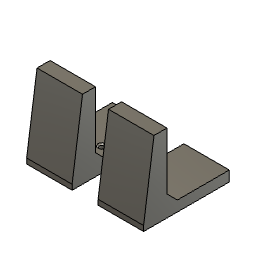
wordclock_standfuss_v2 (Autodesk Fusion 360 design; units mm, degrees)
Autodesk Fusion 360 part; units mm, degrees
other "Grundnetzelement1"
sketch "Skizze1" plane through (20, 30, 0) normal (1, 0, 0) x (0, 1, 0)
other "Netzschnitt1"
sketch "Skizze2" plane through (-10, 30, 0) normal (1, 0, 0) x (0, 1, 0)
  line L0 (-30, 33) -> (-26, 33)
  line L1 (-26, 33) -> (-26, -33)
  line L2 (-26, -33) -> (-30, -33)
  line L3 (-30, -33) -> (-30, 33)
  line L4 (-26, 15) -> (30, 15)
  line L5 (30, 15) -> (30, 25)
  line L6 (30, 25) -> (-26, 25)
  line L7 (-26, 25) -> (-26, 15)
  line L8 (30, 25) -> (-26, 33)
  line L9 (-26, 33) -> (-27.26, 24.18)
  line L10 (-27.26, 24.18) -> (28.74, 16.18)
  line L11 (28.74, 16.18) -> (30, 25)
  constraint horizontal L0
  constraint vertical L1
  constraint horizontal L2
  constraint vertical L3
  constraint horizontal L4
  constraint vertical L5
  constraint horizontal L6
  constraint vertical L7
  constraint coincident L1 L4.start
  constraint perpendicular L8 L9
  constraint parallel L8 L10
  constraint parallel L9 L11
other "Netzschnitt2"
sketch "Skizze3" plane through (-10, 1, 0) normal (0, 1, 0) x (-1, 0, 0)
  circle A0 centre (-10, 0) radius 2
other "Netzschnitt3"
extrude "Extrusion1" add sketch "Skizze2" along normal blind 20 makes body 1
extrude "Extrusion2" add 1 faces at (-10, 22.6667, 24.3333) along direction (-1, 0, 0) blind 20 on bodies 1 bodies 1
extrude "Extrusion3" cut sketch "Skizze3" along normal blind 4 bodies 1
extrude "Extrusion4" cut 1 faces at (-0.6006, 1, 0.0905) along direction (0, -1, 0) blind 9 on bodies 1 bodies 1
extrude "Extrusion5" add 1 faces at (-20.637, 4, -6.1965) along direction (0, 1, 0) blind 4 on bodies 1 bodies 1
chamfer "Fase1" distance 8 angle 45 1 edges at (-10, 8, 15) on bodies 1
chamfer "Fase2" distance 1 angle 45 1 edges at (1.8647, 8, 0.7232) on bodies 1
extrude "Extrusion6" cut 1 faces at (-30, 26.6667, 24.3333) along direction (1, 0, 0) blind 5 on bodies 1 bodies 1
ref_plane "Arbeitsebene1" through (20, 30, 0) normal (1, 0, 0) x (0, 0, -1)
mirror "Spiegeln1" about plane through (20, 30, 0) normal (1, 0, 0) of bodies 1 makes body 2
copy_body "Körper->Berechn1" bodies 2 removing the originals makes body 3 in component "standfuss_v2_mirrored"
copy_body "Körper->Berechn2" bodies 1 removing the originals makes body 4 in component "standfuss_v2_normal"
component "standfuss_v2_mirrored" placed x (1, 0, 0) y (0, 1, 0) z (0, 0, 1) at (0, 0, 0)
component "standfuss_v2_normal" placed x (1, 0, 0) y (0, 1, 0) z (0, 0, 1) at (0, 0, 0)
named bodies: "standfuss_v2_normal", "standfuss_v2_mirrored"
